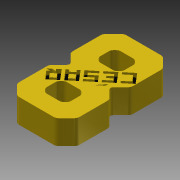
# Autodesk Inventor part: Part1
Saved by Autodesk Inventor 2014 (Build 180170000, 170)
## iProperties
Created: 2015-08-08
Part Number: Part1
Material: Generic
Document SubType Name: Modeling
Designer: Rubén
Density: 1 g/cm^3
Appearance: Glossy - Gold
Author: Rubén
Autodesk Inventor part; units mm, degrees
ref_plane "YZ Plane" through (0, 0, 0) normal (1, 0, 0) x (0, 1, 0)
ref_plane "XZ Plane" through (0, 0, 0) normal (0, 1, 0) x (-1, 0, 0)
ref_plane "XY Plane" through (0, 0, 0) normal (0, 0, 1) x (1, 0, 0)
sketch "Sketch1" plane through (0, 0, 0) normal (0, 1, 0) x (-1, 0, 0)
  line L0 (0, 0) -> (0, 38.5027) construction
  line L1 (0, 38.5027) -> (-13.5, 27.1748) construction
  line L2 (-13.5, 27.1748) -> (-13.5, 50.6722) construction
  line L3 (-13.5, 50.6722) -> (0, 62) construction
  line L4 (0, 62) -> (18, 62) construction
  line L5 (18, 62) -> (18, 0) construction
  line L6 (18, 0) -> (31.5, 0) construction
  line L7 (31.5, 0) -> (31.5, -18) construction
  line L8 (31.5, -18) -> (-13.5, -18) construction
  line L9 (-13.5, -18) -> (-13.5, 0) construction
  line L10 (-13.5, 0) -> (0, 0) construction
  line L11 (9, 62) -> (9, -18) construction
  line L12 (9, 22) -> (31.5, 22) construction
  line L13 (9, -18) -> (23.5, -18)
  line L14 (23.5, -18) -> (31.5, -10)
  line L15 (23.5, -18) -> (34.8137, -18) construction
  line L16 (31.5, -10) -> (31.5, 14)
  line L17 (31.5, 14) -> (23.5, 22)
  line L18 (9, -18) -> (-5.5, -18)
  line L19 (-5.5, -18) -> (-13.5, -10)
  line L20 (-13.5, -10) -> (-13.5, 14)
  line L21 (-13.5, 14) -> (-5.5, 22)
  line L22 (9, 62) -> (23.5, 62)
  line L23 (23.5, 62) -> (31.5, 54)
  line L24 (31.5, 54) -> (31.5, 30)
  line L25 (31.5, 30) -> (23.5, 22)
  line L26 (-13.5, 30) -> (-5.5, 22)
  line L27 (-13.5, 54) -> (-13.5, 30)
  line L28 (-5.5, 62) -> (-13.5, 54)
  line L29 (9, 62) -> (-5.5, 62)
  line L30 (3, 49.5) -> (15, 49.5)
  line L31 (18, 46.5) -> (18, 37.5)
  line L32 (15, 34.5) -> (3, 34.5)
  line L33 (0, 37.5) -> (0, 46.5)
  line L34 (3, 49.5) -> (0, 46.5)
  line L35 (15, 49.5) -> (18, 46.5)
  line L36 (18, 37.5) -> (15, 34.5)
  line L37 (3, 34.5) -> (0, 37.5)
  line L38 (3, -5.5) -> (15, -5.5)
  line L39 (18, -2.5) -> (18, 6.5)
  line L40 (15, 9.5) -> (3, 9.5)
  line L41 (0, 6.5) -> (0, -2.5)
  line L42 (3, -5.5) -> (0, -2.5)
  line L43 (15, -5.5) -> (18, -2.5)
  line L44 (18, 6.5) -> (15, 9.5)
  line L45 (3, 9.5) -> (0, 6.5)
  line L46 (0, 42) -> (9, 42) construction
  line L47 (-13.5, 42) -> (9, 42) construction
  point P0 (0, 49.5)
  point P1 (18, 34.5)
  point P2 (18, 49.5)
  point P3 (0, 34.5)
  point P4 (0, -5.5)
  point P5 (18, 9.5)
  point P6 (18, -5.5)
  point P7 (0, 9.5)
  dimension "d0" = 50
  dimension "d1" = 80
  dimension "d2" = 18
  dimension "d3" = 18
  dimension "d4" = 13.5
  dimension "d5" = 13.5
  dimension "d6" = 18
  dimension "d7" = 0
  dimension "d8" = 0
  dimension "d9" = 0
  dimension "d47" = 45
  dimension "d48" = 135
  dimension "d49" = 8
  dimension "d50" = 8
  dimension "d51" = 3
  dimension "d52" = 3
  dimension "d53" = 3
  dimension "d54" = 3
  dimension "d55" = 3
  dimension "d56" = 3
  dimension "d57" = 3
  dimension "d58" = 3
  dimension "d59" = 0
  dimension "d60" = 0
  dimension "d61" = 0
  dimension "d62" = 15
  constraints: 96 end point, 22 point on line, 22 symmetric about line, 10 parallel, 5 midpoint, 4 perpendicular, 2 horizontal, 1 collinear, 1 equal length, 1 vertical
  measures "d0" angle of L1 L0
  measures "d1" distance between parallel lines of L8 L4
  measures "d2" distance between parallel lines of L5 L0
  measures "d3" distance of L8.end L9.end
  measures "d4" distance between parallel lines of L0 L9
  measures "d5" distance between parallel lines of L7 L5
  measures "d6" distance between parallel lines of L1 L3
  measures "d7" horizontal distance of L0.end L3.end
  measures "d8" distance between parallel lines of L9 L2
  measures "d9" vertical distance of L0.start L5.end
  measures "d47" angle of L15 L14
  measures "d48" angle of L17 L16
  measures "d49" horizontal distance of L16.end L17.end
  measures "d50" horizontal distance of L14.end L13.end
  measures "d51" distance of L30.start point (0, 49.5)
  measures "d52" distance of L33.end point (0, 49.5)
  measures "d53" distance of L30.end point (18, 49.5)
  measures "d54" distance of L31.start point (18, 49.5)
  measures "d55" distance of L31.end point (18, 34.5)
  measures "d56" distance of L32.start point (18, 34.5)
  measures "d57" distance of L32.end point (0, 34.5)
  measures "d58" distance of L33.start point (0, 34.5)
  measures "d59" distance between parallel lines of L5 L31
  measures "d60" distance between parallel lines of L0 L33
  measures "d61" distance between parallel lines of L47 L46
  measures "d62" distance between parallel lines of L32 L30
extrude "Extrusion1" add sketch "Sketch1" along normal blind 18
fillet "Fillet4" radius 4 12 edges at (5.5, 9, 62) (13.5, 9, 54) (13.5, 9, 30) (13.5, 9, 14) (13.5, 9, -10) (5.5, 9, -18) (-23.5, 9, -18) (-31.5, 9, -10) (-31.5, 9, 14) (-31.5, 9, 30) (-31.5, 9, 54) (-23.5, 9, 62)
fillet "Fillet5" radius 2 2 edges at (5.5, 9, 22) (-23.5, 9, 22)
fillet "Fillet6" radius 3 16 edges at (-15, 9, 49.5) (-18, 9, 46.5) (-3, 9, 49.5) (0, 9, 46.5) (0, 9, 37.5) (-3, 9, 34.5) (-18, 9, 37.5) (-15, 9, 34.5) (-3, 9, -5.5) (-15, 9, -5.5) (-3, 9, 9.5) (0, 9, 6.5) (0, 9, -2.5) (-15, 9, 9.5) (-18, 9, 6.5) (-18, 9, -2.5)
sketch "Sketch2" plane through (0, 18, 0) normal (0, 1, 0) x (1, 0, 0)
  line L0 (13.0478, -10.0332) -> (6.6199, -2.3727)
  line L1 (0.4915, -7.515) -> (6.6199, -2.3727)
  line L2 (13.0478, -10.0332) -> (6.9194, -15.1755)
  line L3 (6.9194, -15.1755) -> (5.6338, -13.6434)
  line L4 (5.6338, -13.6434) -> (10.2301, -9.7867)
  line L5 (10.2301, -9.7867) -> (6.3734, -5.1904)
  line L6 (6.3734, -5.1904) -> (1.7771, -9.0471)
  line L7 (1.7771, -9.0471) -> (0.4915, -7.515)
  line L8 (5.3873, -16.461) -> (-1.0406, -8.8006)
  line L9 (-1.0406, -8.8006) -> (-7.1689, -13.9429)
  line L10 (-5.8833, -15.475) -> (-7.1689, -13.9429)
  line L11 (-5.8833, -15.475) -> (-1.2871, -11.6183)
  line L12 (-1.2871, -11.6183) -> (-0.0015, -13.1504)
  line L13 (-0.0015, -13.1504) -> (-3.0657, -15.7215)
  line L14 (-3.0657, -15.7215) -> (-1.7801, -17.2536)
  line L15 (-1.7801, -17.2536) -> (1.2841, -14.6824)
  line L16 (1.2841, -14.6824) -> (2.5697, -16.2145)
  line L17 (2.5697, -16.2145) -> (-2.0266, -20.0713)
  line L18 (-2.0266, -20.0713) -> (-0.741, -21.6033)
  line L19 (5.3873, -16.461) -> (-0.741, -21.6033)
  line L20 (-2.2731, -22.8889) -> (-6.1298, -18.2927)
  line L21 (-6.1298, -18.2927) -> (-10.7261, -22.1494)
  line L22 (-10.7261, -22.1494) -> (-12.0117, -20.6173)
  line L23 (-12.0117, -20.6173) -> (-7.4154, -16.7606)
  line L24 (-7.4154, -16.7606) -> (-8.701, -15.2285)
  line L25 (-8.701, -15.2285) -> (-14.8294, -20.3708)
  line L26 (-14.8294, -20.3708) -> (-10.9726, -24.967)
  line L27 (-10.9726, -24.967) -> (-6.3764, -21.1103)
  line L28 (-6.3764, -21.1103) -> (-5.0908, -22.6424)
  line L29 (-5.0908, -22.6424) -> (-9.6871, -26.4991)
  line L30 (-9.6871, -26.4991) -> (-8.4015, -28.0312)
  line L31 (-2.2731, -22.8889) -> (-8.4015, -28.0312)
  line L32 (-9.9336, -29.3168) -> (-16.3614, -21.6564)
  line L33 (-22.4898, -26.7987) -> (-16.0619, -34.4591)
  line L34 (-16.0619, -34.4591) -> (-9.9336, -29.3168)
  line L35 (-12.7512, -29.0703) -> (-15.3224, -26.0061)
  line L36 (-17.594, -35.7447) -> (-24.0219, -28.0842)
  line L37 (-1.6672, -26.2967) -> (3.2873, -20.1813)
  line L38 (6.9194, -15.1755) -> (5.3873, -16.461) construction
  line L39 (-0.741, -21.6033) -> (-2.2731, -22.8889) construction
  line L40 (-8.4015, -28.0312) -> (-9.9336, -29.3168) construction
  line L41 (-16.0619, -34.4591) -> (-17.594, -35.7447) construction
  line L42 (-22.4898, -26.7987) -> (-24.0219, -28.0842) construction
  line L43 (0.4915, -7.515) -> (-1.0406, -8.8006) construction
  line L44 (-14.8294, -20.3708) -> (-16.3614, -21.6564) construction
  line L45 (-9.6871, -26.4991) -> (-10.9726, -24.967) construction
  line L46 (-6.1298, -18.2927) -> (-7.4154, -16.7606) construction
  line L47 (-6.3764, -21.1103) -> (-4.8443, -19.8247) construction
  line L48 (-10.7261, -22.1494) -> (-9.4405, -23.6815) construction
  line L49 (-10.7261, -22.1494) -> (-12.2582, -23.435) construction
  line L50 (2.5697, -16.2145) -> (4.1017, -14.929) construction
  line L51 (-17.8935, -22.9419) -> (-16.3614, -21.6564)
  line L52 (-20.9577, -25.5131) -> (-22.4898, -26.7987)
  line L53 (-12.7512, -29.0703) -> (-11.2191, -27.7847) construction
  line L54 (-12.7512, -29.0703) -> (-15.8154, -31.6414)
  line L55 (-15.8154, -31.6414) -> (-17.3475, -32.927) construction
  line L56 (-12.7512, -29.0703) -> (-11.4657, -30.6024) construction
  line L57 (-17.594, -35.7447) -> (-23.7224, -40.887)
  line L58 (-20.4117, -35.4982) -> (-18.8796, -34.2126) construction
  line L59 (-20.4117, -35.4982) -> (-19.1261, -37.0302) construction
  line L60 (-24.0219, -28.0842) -> (-26.32, -30.0126)
  line L61 (-26.32, -30.0126) -> (-25.0344, -31.5447)
  line L62 (-25.0344, -31.5447) -> (-27.8521, -31.2982)
  line L63 (-27.8521, -31.2982) -> (-30.1502, -33.2265)
  line L64 (-30.1502, -33.2265) -> (-27.3326, -33.473)
  line L65 (-27.3326, -33.473) -> (-28.8647, -34.7586)
  line L66 (-28.8647, -34.7586) -> (-23.7224, -40.887)
  line L67 (-22.9828, -32.434) -> (-26.047, -35.0051)
  line L68 (-26.047, -35.0051) -> (-23.4759, -38.0693)
  line L69 (-23.4759, -38.0693) -> (-20.4117, -35.4982)
  line L70 (3.2873, -20.1813) -> (2.929, -22.44)
  line L71 (-28.8647, -34.7586) -> (-30.1502, -33.2265) construction
  line L72 (-26.32, -30.0126) -> (-27.8521, -31.2982) construction
  line L73 (-20.4117, -35.4982) -> (-22.9828, -32.434)
  line L74 (-26.047, -35.0051) -> (-27.3326, -33.473) construction
  line L75 (-7.1689, -13.9429) -> (-8.701, -15.2285) construction
  line L76 (2.929, -22.44) -> (-1.6672, -26.2967)
  line L77 (2.929, -22.44) -> (4.2515, -21.3303) construction
  line L78 (4.2515, -21.3303) -> (3.2873, -20.1813) construction
  line L79 (3.2873, -20.1813) -> (2.3231, -19.0322) construction
  line L80 (-4.2426, -9.5) -> (-13.7574, -9.5) projected
  line L81 (-13.7574, -34.5) -> (-4.2426, -34.5) projected
  line L82 (-15.3224, -26.0061) -> (-18.3866, -28.5773)
  line L83 (-15.8154, -31.6414) -> (-18.3866, -28.5773)
  line L84 (-19.6721, -27.0452) -> (-20.9577, -25.5131)
  line L85 (-15.3224, -26.0061) -> (-16.608, -24.474) construction
  line L86 (-16.608, -24.474) -> (-17.8935, -22.9419)
  line L87 (-16.608, -24.474) -> (-19.6721, -27.0452)
  line L88 (-5.3373, -25.4601) -> (-11.7652, -17.7996) construction
  line L89 (-8.5627, -34.5) -> (-8.5627, -9.5) construction
  line L90 (9.8338, -6.2029) -> (-26.9363, -37.0568) construction
  point P0 (0, 0)
  dimension "d18" = 10
  dimension "d19" = 8
  dimension "d20" = 2
  dimension "d21" = 45
  dimension "d26" = 0
  dimension "d29" = 3
  dimension "d31" = 30
  dimension "d67" = 40
  constraints: 178 end point, 42 equal length, 42 perpendicular, 23 parallel, 20 collinear, 14 point on line, 4 midpoint
  measures "d18" distance of L0.start L0.end
  measures "d19" distance of L0.start L2.end
  measures "d20" distance between parallel lines of L18 L14
  measures "d21" angle of L61 L62
  measures "d26" distance from line of L65 L61.end
  measures "d29" distance between parallel lines of L19 L76
  measures "d31" angle of L37 L70
  measures "d67" angle of L80 L25
extrude "Extrusion2" cut sketch "Sketch2" against normal blind 3
body "Solid1"
